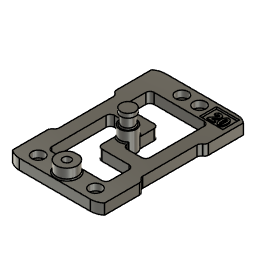
FS40 Unified Adapter 2MPix v1 (Autodesk Fusion 360 design; units mm, degrees)
Autodesk Fusion 360 part; units mm, degrees
note: some values were not read from the file. Set by a fixed rule: which sketch regions a step uses.
sketch "Schizzo5" plane through (0, 0, 0) normal (0, 0, 1) x (1, 0, 0)
  line L0 (334.1836, 79.5632) -> (384.1836, 79.5632) construction
  line L1 (384.1836, 79.5632) -> (384.1836, 9.5632) construction
  line L2 (384.1836, 9.5632) -> (334.1836, 9.5632) construction
  line L3 (334.1836, 9.5632) -> (334.1836, 79.5632) construction
  circle A0 centre (342.1836, 17.5632) radius 8
  circle A1 centre (342.1836, 71.5632) radius 8
  line L4 (359.1836, 79.5632) -> (359.1836, 9.5632) construction
  circle A2 centre (376.1836, 71.5632) radius 8
  circle A3 centre (376.1836, 17.5632) radius 8
  line L5 (334.1836, 74.5632) -> (384.1836, 74.5632) construction
  line L6 (334.1836, 15.3132) -> (384.1836, 15.3132) construction
  circle A4 centre (359.1836, 15.3132) radius 1.9
  line L7 (345.4836, 79.5632) -> (345.4836, 9.5632) construction
  line L8 (372.8836, 79.5632) -> (372.8836, 9.5632) construction
  circle A5 centre (345.4836, 15.3132) radius 1.6
  circle A6 centre (345.4836, 15.3132) radius 3
  line L9 (354.9536, 79.5632) -> (354.9536, 9.5632) construction
  line L10 (363.4136, 79.5632) -> (363.4136, 9.5632) construction
  circle A7 centre (354.9536, 74.5632) radius 1.6
  circle A8 centre (354.9536, 74.5632) radius 3
  circle A9 centre (363.4136, 74.5632) radius 3
  circle A10 centre (363.4136, 74.5632) radius 1.6
  circle A11 centre (372.8836, 15.3132) radius 3
  circle A12 centre (372.8836, 15.3132) radius 1.6
  line L11 (334.1836, 44.3132) -> (384.1836, 44.3132) construction
  circle A13 centre (359.1836, 44.5632) radius 2.9
  line L12 (334.1836, 71.5632) -> (334.1836, 17.5632)
  line L13 (342.1836, 9.5632) -> (376.1836, 9.5632)
  line L14 (384.1836, 17.5632) -> (384.1836, 71.5632)
  line L15 (376.1836, 79.5632) -> (342.1836, 79.5632)
  circle A14 centre (359.1836, 44.5632) radius 4
  circle A15 centre (359.1836, 15.3132) radius 5
  dimension "d289" = 50
  dimension "d290" = 70
  dimension "d291" = 8
  dimension "d292" = 8
  dimension "d293" = 5
  dimension "d294" = 59.25
  dimension "d295" = 3.8
  dimension "d296" = 38.7
  dimension "d297" = 38.7
  dimension "d298" = 3.2
  dimension "d299" = 6
  dimension "d300" = 29.23
  dimension "d301" = 29.23
  dimension "d302" = 3.2
  dimension "d303" = 6
  dimension "d304" = 29
  dimension "d305" = 5.8
  dimension "d386" = 8
  dimension "d393" = 10
  constraint horizontal L0
  constraint vertical L1
  constraint horizontal L2
  constraint vertical L3
  constraint tangent L3 A0
  constraint tangent L2 A0
  constraint tangent L0 A1
  constraint tangent L3 A1
  constraint midpoint L0 L4.start
  constraint midpoint L2 L4.end
  constraint symmetric A0 L4 A3
  constraint symmetric A1 L4 A2
  constraint coincident L3 L5.start
  constraint coincident L1 L5.end
  constraint perpendicular L1 L5
  constraint coincident L3 L6.start
  constraint coincident L1 L6.end
  constraint perpendicular L1 L6
  constraint midpoint L6 A4.centre
  constraint coincident L0 L7.start
  constraint coincident L2 L7.end
  constraint perpendicular L2 L7
  constraint coincident L0 L8.start
  constraint coincident L2 L8.end
  constraint perpendicular L2 L8
  constraint coincident L7 A5.centre
  constraint coincident L6 A5.centre
  constraint concentric A5 A6
  constraint coincident L0 L9.start
  constraint coincident L2 L9.end
  constraint perpendicular L2 L9
  constraint coincident L0 L10.start
  constraint coincident L2 L10.end
  constraint perpendicular L2 L10
  constraint coincident L5 A7.centre
  constraint coincident L9 A7.centre
  constraint concentric A7 A8
  constraint symmetric L4 A5 A12
  constraint symmetric L4 A6 A11
  constraint symmetric L4 A7 A10
  constraint symmetric L4 A8 A9
  constraint coincident L3 L11.start
  constraint coincident L1 L11.end
  constraint perpendicular L1 L11
  constraint midpoint L4 A13.centre
  constraint coincident A1 L12.start
  constraint coincident L3 L12.start
  constraint coincident L3 L12.end
  constraint coincident A0 L12.end
  constraint coincident A0 L13.start
  constraint coincident L2 L13.start
  constraint coincident A3 L13.end
  constraint coincident L2 L13.end
  constraint coincident A3 L14.start
  constraint coincident L1 L14.start
  constraint coincident A2 L14.end
  constraint coincident L1 L14.end
  constraint coincident A2 L15.start
  constraint coincident L0 L15.start
  constraint coincident L0 L15.end
  constraint coincident A1 L15.end
  constraint concentric A13 A14
  constraint concentric A4 A15
  measures "d289" distance of L0.start L0.end
  measures "d290" distance of L0.start L2.end
  measures "d291" radius of A0
  measures "d292" radius of A1
  measures "d293" distance of L0 L5
  measures "d294" distance of L5 L6
  measures "d295" diameter of A4
  measures "d296" distance of L1 L7
  measures "d297" distance of L3 L8
  measures "d298" diameter of A5
  measures "d299" diameter of A6
  measures "d300" distance of L1 L9
  measures "d301" distance of L3 L10
  measures "d302" diameter of A7
  measures "d303" diameter of A8
  measures "d304" distance of L6 L11
  measures "d305" diameter of A13
  measures "d386" diameter of A14
  measures "d393" diameter of A15
extrude "Estrusione26" add sketch "Schizzo5" along normal blind 5 contours A0 | A0 A1 A2 A3 L12 L13 L14 L15 | A1 | A3 | A2 | A6 | A8 | A9 | A11 | A14 | A15
extrude "Estrusione27" cut sketch "Schizzo5" against normal blind 3.2 from surface at 5 contours A6 | A8 | A9 | A11
extrude "Estrusione34" add sketch "Schizzo5" along normal blind 10 contours A15
sketch "Schizzo16" plane through (0, 0, 5) normal (0, 0, 1) x (-1, 0, 0)
  circle A0 centre (-363.4136, -74.5632) radius 3
  circle A1 centre (-345.4836, -15.3132) radius 3
  circle A2 centre (-354.9536, -74.5632) radius 3
  circle A3 centre (-372.8836, -15.3132) radius 3
  circle A4 centre (-359.1836, -44.5632) radius 2.9
  line L0 (-376.1836, -79.5632) -> (-342.1836, -79.5632)
  arc A5 (-342.1836, -79.5632) -> (-334.1836, -71.5632) centre (-342.1836, -71.5632) ccw
  line L1 (-334.1836, -71.5632) -> (-334.1836, -17.5632)
  arc A6 (-334.1836, -17.5632) -> (-342.1836, -9.5632) centre (-342.1836, -17.5632) ccw
  line L2 (-342.1836, -9.5632) -> (-376.1836, -9.5632)
  arc A7 (-376.1836, -9.5632) -> (-384.1836, -17.5632) centre (-376.1836, -17.5632) ccw
  line L3 (-384.1836, -17.5632) -> (-384.1836, -71.5632)
  arc A8 (-384.1836, -71.5632) -> (-376.1836, -79.5632) centre (-376.1836, -71.5632) ccw
  line L4 (-334.1836, -79.5632) -> (-384.1836, -79.5632) construction
  line L5 (-384.1836, -79.5632) -> (-384.1836, -9.5632) construction
  line L6 (-384.1836, -9.5632) -> (-334.1836, -9.5632) construction
  line L7 (-334.1836, -9.5632) -> (-334.1836, -79.5632) construction
  line L8 (-359.1836, -79.5632) -> (-359.1836, -9.5632) construction
  line L9 (-373.1836, -56.0632) -> (-345.1836, -56.0632)
  line L10 (-345.1836, -56.0632) -> (-345.1836, -69.0632)
  line L11 (-345.1836, -69.0632) -> (-373.1836, -69.0632)
  line L12 (-373.1836, -69.0632) -> (-373.1836, -56.0632)
  line L13 (-373.1836, -56.0632) -> (-345.1836, -69.0632) construction
  line L14 (-345.1836, -56.0632) -> (-373.1836, -69.0632) construction
  line L15 (-373.1836, -20.0632) -> (-345.1836, -20.0632)
  line L16 (-345.1836, -20.0632) -> (-345.1836, -33.0632)
  line L17 (-345.1836, -33.0632) -> (-373.1836, -33.0632)
  line L18 (-373.1836, -33.0632) -> (-373.1836, -20.0632)
  line L19 (-373.1836, -20.0632) -> (-345.1836, -33.0632) construction
  line L20 (-345.1836, -20.0632) -> (-373.1836, -33.0632) construction
  line L21 (-345.1836, -50.0632) -> (-356.1836, -50.0632)
  line L22 (-356.1836, -50.0632) -> (-356.1836, -33.0632)
  line L23 (-356.1836, -33.0632) -> (-345.1836, -33.0632)
  line L24 (-345.1836, -33.0632) -> (-345.1836, -50.0632)
  line L25 (-334.1836, -79.5632) -> (-337.1836, -79.5632)
  line L26 (-337.1836, -79.5632) -> (-337.1836, -9.5632)
  line L27 (-337.1836, -9.5632) -> (-334.1836, -9.5632)
  line L28 (-334.1836, -9.5632) -> (-334.1836, -79.5632)
  line L29 (-381.1836, -79.5632) -> (-381.1836, -9.5632)
  line L30 (-362.1836, -33.0632) -> (-373.1836, -33.0632)
  line L31 (-362.1836, -56.0632) -> (-373.1836, -56.0632)
  line L32 (-373.1836, -56.0632) -> (-373.1836, -39.0632)
  line L33 (-373.1836, -39.0632) -> (-362.1836, -39.0632)
  line L34 (-362.1836, -39.0632) -> (-362.1836, -56.0632)
  line L35 (-334.1836, -44.5632) -> (-384.1836, -44.5632) construction
  line L36 (-339.1836, -29.5632) -> (-337.1836, -29.5632)
  line L37 (-337.1836, -29.5632) -> (-337.1836, -59.5632)
  line L38 (-337.1836, -59.5632) -> (-339.1836, -59.5632)
  line L39 (-339.1836, -59.5632) -> (-339.1836, -29.5632)
  line L40 (-339.1836, -29.5632) -> (-337.1836, -59.5632) construction
  line L41 (-337.1836, -29.5632) -> (-339.1836, -59.5632) construction
  line L42 (-379.1836, -59.5632) -> (-379.1836, -29.5632)
  line L43 (-381.1836, -59.5632) -> (-379.1836, -59.5632)
  line L44 (-381.1836, -29.5632) -> (-381.1836, -59.5632)
  line L45 (-379.1836, -29.5632) -> (-381.1836, -29.5632)
  line L46 (-368, -78.0632) -> (-379, -78.0632)
  line L47 (-379, -78.0632) -> (-379, -70.0632)
  line L48 (-379, -70.0632) -> (-368, -70.0632)
  line L49 (-368, -70.0632) -> (-368, -78.0632)
  circle A9 centre (-359.1836, -15.3132) radius 5
  point P0 (-359.1836, -62.5632)
  point P1 (-359.1836, -26.5632)
  point P2 (-338.1836, -44.5632)
  dimension "d311" = 28
  dimension "d312" = 13
  dimension "d313" = 17
  dimension "d314" = 28
  dimension "d315" = 13
  dimension "d316" = 17
  dimension "d335" = 3
  dimension "d366" = 2
  dimension "d367" = 30
  dimension "d375" = 17
  dimension "d376" = 11
  dimension "d385" = 1.5
  constraint horizontal L4
  constraint vertical L5
  constraint horizontal L6
  constraint vertical L7
  constraint collinear L0 L4
  constraint collinear L2 L6
  constraint collinear L1 L7
  constraint collinear L3 L5
  constraint midpoint L4 L8.start
  constraint midpoint L6 L8.end
  constraint horizontal L9
  constraint perpendicular L9 L10
  constraint parallel L9 L11
  constraint parallel L10 L12
  constraint coincident L13 P0
  constraint coincident L14 P0
  constraint coincident L8 P0
  constraint horizontal L15
  constraint perpendicular L15 L16
  constraint parallel L15 L17
  constraint parallel L16 L18
  constraint coincident L19 P1
  constraint coincident L20 P1
  constraint coincident L8 P1
  constraint horizontal L21
  constraint vertical L22
  constraint horizontal L23
  constraint vertical L24
  constraint collinear L17 L23
  constraint collinear L16 L24
  constraint horizontal L25
  constraint vertical L26
  constraint horizontal L27
  constraint vertical L28
  constraint collinear L7 L28
  constraint collinear L4 L25
  constraint collinear L6 L27
  constraint symmetric L8 L25.end L29.start
  constraint symmetric L8 L26.end L29.end
  constraint symmetric L8 L22.end L30.start
  constraint symmetric L8 L16.end L17.end
  constraint horizontal L31
  constraint vertical L32
  constraint horizontal L33
  constraint vertical L34
  constraint coincident L9.start L12.end
  constraint equal L21 L33
  constraint equal L22 L34
  constraint midpoint L7 L35.start
  constraint midpoint L5 L35.end
  constraint horizontal L36
  constraint perpendicular L36 L37
  constraint parallel L36 L38
  constraint parallel L37 L39
  constraint coincident L40 P2
  constraint coincident L41 P2
  constraint coincident L35 P2
  constraint collinear L26 L37
  constraint symmetric L8 L36.start L42.end
  constraint symmetric L8 L36.end L44.start
  constraint symmetric L8 L37.end L43.start
  constraint symmetric L8 L38.end L42.start
  constraint horizontal L46
  constraint vertical L47
  constraint horizontal L48
  constraint vertical L49
  measures "d311" distance of L10.end L11.end
  measures "d312" distance of L9.end L10.end
  measures "d313" distance of L4 P0
  measures "d314" distance of L16.end L17.end
  measures "d315" distance of L15.end L16.end
  measures "d316" distance of L6 P1
  measures "d335" distance of L26 L28
  measures "d366" distance of L37.end L38.end
  measures "d367" distance of L36.end L37.end
  measures "d375" distance of L17 L21
  measures "d376" distance of L32 L34
  measures "d385" distance of L4 L46
extrude "Estrusione28" cut sketch "Schizzo16" against normal blind 5 contours A7 L3 A8 L29 L44 | A5 L1 A6 L26 L28 L37 | L29 L42 L43 L44 L45 | L26 L36 L37 L38 L39 | L9 L31 L32 L33 L34 | L9 L10 L11 L12 L31 | L15 L16 L17 L18 L23 L30 A9 | L15 A9 | L17 L21 L22 L23 L24 picked at (-358.8679, -20.1163)
extrude "Estrusione35" cut sketch "Schizzo16" along normal mid plane 10 contours L15 A9 picked at (-358.8679, -20.1163)
fillet "Raccordo10" radius 0.5 1 edges at (359.1836, 10.3132, 5)
fillet "Raccordo1" radius 2 1 edges at (356.1836, 50.0632, 2.5)
fillet "Raccordo1" radius 2 1 edges at (345.1836, 50.0632, 2.5)
fillet "Raccordo1" radius 2 1 edges at (356.1836, 33.0632, 2.5)
fillet "Raccordo2" radius 2 1 edges at (345.1836, 69.0632, 2.5)
fillet "Raccordo2" radius 2 1 edges at (373.1836, 69.0632, 2.5)
fillet "Raccordo2" radius 2 1 edges at (373.1836, 33.0632, 2.5)
fillet "Raccordo2" radius 2 1 edges at (345.1836, 20.0632, 2.5)
fillet "Raccordo2" radius 2 1 edges at (373.1836, 20.0632, 2.5)
fillet "Raccordo3" radius 2 1 edges at (345.1836, 56.0632, 2.5)
fillet "Raccordo3" radius 2 1 edges at (362.1836, 56.0632, 2.5)
fillet "Raccordo3" radius 2 2 edges at (362.1836, 39.0632, 2.5) (373.1836, 39.0632, 2.5)
extrude "Estrusione29" add sketch "Schizzo5" along normal blind 15 contours A13
extrude "Estrusione33" add sketch "Schizzo5" along normal blind 10 contours A14
fillet "Raccordo8" radius 0.5 2 edges at (359.1836, 48.5632, 5) (359.1836, 40.5632, 5)
fillet "Raccordo8" radius 0.5 1 edges at (356.4798, 43.5145, 10)
sketch "Schizzo17" plane through (0, 0, 15) normal (0, 0, 1) x (-1, 0, 0)
  circle A0 centre (-359.1836, -44.5632) radius 2.9
  line L0 (-356.2836, -47.4632) -> (-362.0836, -47.4632) construction
  line L1 (-362.0836, -47.4632) -> (-362.0836, -41.6632) construction
  line L2 (-362.0836, -41.6632) -> (-356.2836, -41.6632) construction
  line L3 (-356.2836, -41.6632) -> (-356.2836, -47.4632) construction
  line L4 (-356.2836, -44.5632) -> (-362.0836, -44.5632) construction
  line L5 (-359.1836, -47.4632) -> (-359.1836, -41.6632) construction
  circle A1 centre (-359.1836, -44.5632) radius 3.5
  dimension "d372" = 7
  constraint horizontal L0
  constraint vertical L1
  constraint horizontal L2
  constraint vertical L3
  constraint tangent A0 L0
  constraint tangent A0 L3
  constraint tangent A0 L2
  constraint tangent A0 L1
  constraint midpoint L3 L4.start
  constraint midpoint L1 L4.end
  constraint midpoint L0 L5.start
  constraint midpoint L2 L5.end
  constraint concentric A0 A1
  measures "d372" diameter of A1
extrude "Estrusione30" add sketch "Schizzo17" along normal blind 2 contours A0 | A1
fillet "Raccordo5" radius 2 4 edges at (337.1836, 59.5632, 2.5) (339.1836, 59.5632, 2.5) (337.1836, 29.5632, 2.5) (339.1836, 29.5632, 2.5)
fillet "Raccordo6" radius 2 4 edges at (381.1836, 29.5632, 2.5) (379.1836, 29.5632, 2.5) (381.1836, 59.5632, 2.5) (379.1836, 59.5632, 2.5)
extrude "Estrusione31" cut sketch "Schizzo16" against normal blind 1 contours L46 L47 L48 L49
sketch "Schizzo19" plane through (0, 0, 4) normal (0, 0, 1) x (-1, 0, 0)
  line L0 (-368, -70.0632) -> (-379, -70.0632)
  line L1 (-379, -70.0632) -> (-379, -78.0632)
  line L2 (-379, -78.0632) -> (-368, -78.0632)
  line L3 (-368, -78.0632) -> (-368, -70.0632)
  line L4 (-368, -70.0632) -> (-379, -70.0632) construction
  line L5 (-379, -70.0632) -> (-379, -78.0632) construction
  line L6 (-379, -78.0632) -> (-368, -78.0632) construction
  line L7 (-368, -78.0632) -> (-368, -70.0632) construction
  dimension "d380" = 5
  text T0 "20" font "Arial" height 5 bold align centre middle in box 11 x 8 at (-368, -70.0632) x (-1, 0) y (0, -1) spacing 1
  constraint coincident L0.end
  constraint coincident L2.end
extrude "Estrusione32" add sketch "Schizzo19" along normal blind 0.5 text T0
equation "d315 = d312"
equation "d316 = d313"
named bodies: "Adattatore V2"
